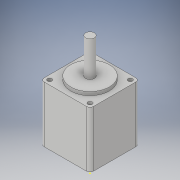
# Autodesk Inventor part: NEMA11
Saved by Autodesk Inventor 2017 (Build 210142000, 142)
## iProperties
Created: 2017-06-15
Part Number: NEMA11
Material: Generic
Document SubType Name: Modeling
Designer: millerid
Density: 1 g/cm^3
Appearance: Default
Author: millerid
Autodesk Inventor part; units mm, degrees
ref_plane "YZ Plane" through (0, 0, 0) normal (1, 0, 0) x (0, 1, 0)
ref_plane "XZ Plane" through (0, 0, 0) normal (0, 1, 0) x (-1, 0, 0)
ref_plane "XY Plane" through (0, 0, 0) normal (0, 0, 1) x (1, 0, 0)
sketch "Sketch1" plane through (0, 0, 0) normal (0, 1, 0) x (-1, 0, 0)
  point P0 (0, 0)
sketch "Sketch2" plane through (0, 0, 0) normal (0, 1, 0) x (-1, 0, 0)
  line L0 (0, 0) -> (28.2, 0)
  line L1 (28.2, 0) -> (28.2, -28.2)
  line L2 (28.2, -28.2) -> (0, -28.2)
  line L3 (0, -28.2) -> (0, 0)
  dimension "d0" = 28.2
  dimension "d1" = 28.2
  constraints: 8 end point, 2 parallel, 1 horizontal, 1 perpendicular
  measures "d0" distance of L1.end L2.end
  measures "d1" distance of L0.end L1.end
extrude "Extrusion1" add sketch "Sketch2" along normal blind 32
sketch "Sketch3" plane through (0, 32, 0) normal (0, 1, 0) x (1, 0, 0)
  circle A0 centre (-14.1, 14.1) radius 11
  point P0 (0, 0)
  dimension "d4" = 22
  constraints: 1 centre point, 1 coincident
  measures "d4" diameter of A0
extrude "Extrusion2" add sketch "Sketch3" along normal blind 2
sketch "Sketch4" plane through (-14.1, 34, -14.1) normal (0, 1, 0) x (1, 0, 0)
  circle A0 centre (0, 0) radius 2.5
  point P0 (14.1, -14.1)
  dimension "d7" = 5
  constraints: 1 centre point
  measures "d7" diameter of A0
extrude "Extrusion3" add sketch "Sketch4" along normal blind 20
sketch "Sketch5" plane through (0, 32, 0) normal (0, 1, 0) x (1, 0, 0)
  circle A0 centre (-25.6, 2.6) radius 1.25
  line L0 (-28.2, 28.2) -> (-28.2, 0) projected
  line L1 (-28.2, 0) -> (0, 0) projected
  circle A1 centre (-25.6, 25.6) radius 1.25
  circle A2 centre (-2.6, 2.6) radius 1.25
  circle A3 centre (-2.6, 25.6) radius 1.25
  dimension "d10" = 2.5
  dimension "d11" = 2.6
  dimension "d12" = 2.6
  dimension "d13" = 2.5
  dimension "d14" = 23
  dimension "d15" = 2.5
  dimension "d16" = 23
  dimension "d17" = 2.5
  constraints: 4 centre point
  measures "d10" diameter of A0
  measures "d11" distance from line of A0.centre L0
  measures "d12" distance from line of A0.centre L1
  measures "d13" diameter of A1
  measures "d14" distance of A1.centre A0.centre
  measures "d15" diameter of A2
  measures "d16" distance of A2.centre A0.centre
  measures "d17" diameter of A3
extrude "Extrusion4" cut sketch "Sketch5" against normal through all
fillet "Fillet1" radius 2 4 edges at (0, 16, 0) (0, 16, -28.2) (-28.2, 16, -28.2) (-28.2, 16, 0)
body "Solid1"
